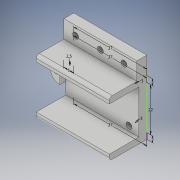
# Autodesk Inventor part: motor_grip_R
Saved by Autodesk Inventor 2019 (Build 230136000, 136)
## iProperties
Created: 2019-04-06
Part Number: motor_grip_R
Material: Ogólny
Document SubType Name: Modeling
Designer: terg
Density: 1 g/cm^3
Appearance: Domyślna
Author: terg
Autodesk Inventor part; units mm, degrees
ref_plane "YZ Plane" through (0, 0, 0) normal (1, 0, 0) x (0, 1, 0)
ref_plane "XZ Plane" through (0, 0, 0) normal (0, 1, 0) x (-1, 0, 0)
ref_plane "XY Plane" through (0, 0, 0) normal (0, 0, 1) x (1, 0, 0)
sketch "Szkic1" plane through (0, 0, 0) normal (0, 0, 1) x (1, 0, 0)
  line L0 (0, 0) -> (37, 0)
  line L1 (37, 0) -> (37, 22)
  line L2 (37, 22) -> (0, 22)
  line L3 (0, 11) -> (-5, 11) construction
  circle A0 centre (-2, 11) radius 1.25
  arc A1 (0, 16) -> (0, 6) centre (0, 11) ccw
  line L4 (37, 22) -> (32, 22) construction
  line L5 (37, 22) -> (37, 19.5) construction
  circle A2 centre (32, 19.5) radius 1.5
  line L6 (37, 0) -> (32, 0) construction
  line L7 (32, 0) -> (32, 2.5) construction
  circle A3 centre (32, 2.5) radius 1.5
  line L8 (0, 22) -> (37, 22)
  line L9 (37, 22) -> (37, 25)
  line L10 (37, 25) -> (0, 25)
  line L11 (0, 25) -> (0, 22)
  line L12 (0, 0) -> (37, 0)
  line L13 (37, 0) -> (37, -3)
  line L14 (37, -3) -> (0, -3)
  line L15 (0, -3) -> (0, 0)
  line L16 (0, 22) -> (0, 16)
  line L17 (0, 6) -> (0, 0)
  dimension "d0" = 37
  dimension "d1" = 22
  dimension "d2" = 5
  dimension "d3" = 2.5
  dimension "d7" = 3
  dimension "d10" = 3
  dimension "d11" = 37
  dimension "d12" = 3
  dimension "d13" = 37
  dimension "d14" = 3
  constraints: 36 end point, 6 equal length, 4 centre point, 4 coincident, 4 horizontal, 4 perpendicular, 4 point on line, 3 point on circle, 1 vertical
  measures "d0" distance of L2.end L1.end
  measures "d1" distance of L1.end L0.end
  measures "d2" distance of L3.start L3.end
  measures "d3" diameter of A0
  measures "d7" diameter of A2
  measures "d10" diameter of A3
  measures "d11" distance of L10.end L9.end
  measures "d12" distance of L9.end L8.end
  measures "d13" distance of L13.end L14.end
  measures "d14" distance of L12.end L13.end
extrude "Wyciągnięcie proste1" add sketch "Szkic1" along normal blind 4 contours L17 A1 L16 L2 L1 L0
sketch "Szkic2" plane through (0, 0, 4) normal (0, 0, 1) x (1, 0, 0)
  circle A0 centre (-2, 11) radius 1.25 projected
  arc A1 (0, 16) -> (0, 6) centre (0, 11) ccw projected
  line L0 (0, 6) -> (0, 0) projected
  line L1 (0, 16) -> (0, 6)
  constraints: 2 end point, 1 vertical
extrude "Wyciągnięcie proste2" add sketch "Szkic2" along normal blind 3
extrude "Wyciągnięcie proste3" add sketch "Szkic1" along normal blind 19 contours L0 L13 L14 L15
extrude "Wyciągnięcie proste4" add sketch "Szkic1" along normal blind 19 contours L2 L11 L10 L9
fillet "Zaokrąglenie2" radius 1.5 1 edges at (18.5, 25, 19)
fillet "Zaokrąglenie3" radius 1.5 1 edges at (18.5, -3, 19)
sketch "Szkic3" plane through (0, 25, 0) normal (0, 1, 0) x (1, 0, 0)
  line L0 (37, -17.5) -> (0, -17.5) projected
  line L1 (37, 0) -> (37, -17.5) projected
  line L2 (37, 0) -> (0, 0) projected
  line L3 (0, 0) -> (0, -17.5) projected
  line L4 (-5, 0) -> (0, 0) projected
  line L5 (0, 0) -> (37, 0)
  line L6 (37, 0) -> (37, -5)
  line L7 (37, -5) -> (0, -5)
  line L8 (0, -5) -> (0, 0)
  dimension "d26" = 37
  dimension "d27" = 5
  constraints: 8 end point, 2 parallel, 1 horizontal, 1 perpendicular
  measures "d26" distance of L6.end L7.end
  measures "d27" distance of L5.end L6.end
extrude "Wyciągnięcie proste5" add sketch "Szkic3" along normal blind 9 contours L7 L3 L2 L1
sketch "Szkic4" plane through (0, 25, 5) normal (0, 0, 1) x (1, 0, 0)
  line L0 (0, 9) -> (0, 0)
  line L1 (0, 0) -> (0, 4.5)
  line L2 (37, 0) -> (37, 9) projected
  circle A0 centre (6, 4.5) radius 1.5
  circle A1 centre (18.5, 4.5) radius 1.5
  circle A2 centre (30.5, 4.5) radius 1.5
  point P0 (0, -25)
  dimension "d30" = 3
  dimension "d31" = 3
  dimension "d32" = 3
  constraints: 4 coincident, 4 end point, 3 centre point, 1 midpoint, 1 vertical
  measures "d30" diameter of A0
  measures "d31" diameter of A1
  measures "d32" diameter of A2
extrude "Wyciągnięcie proste6" cut sketch "Szkic4" against normal blind 9
